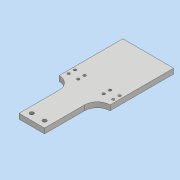
# Autodesk Inventor part: Wspornik pionowy osi Y
Saved by Autodesk Inventor 2018 (Build 220112000, 112)
## iProperties
Created: 2019-01-25
Part Number: Wspornik pionowy osi Y
Material: Ogólny
Document SubType Name: Modeling
Designer: Dawid
Density: 1 g/cm^3
Appearance: Domyślna
Author: Dawid
Autodesk Inventor part; units mm, degrees
ref_plane "YZ Plane" through (0, 0, 0) normal (1, 0, 0) x (0, 1, 0)
ref_plane "XZ Plane" through (0, 0, 0) normal (0, 1, 0) x (-1, 0, 0)
ref_plane "XY Plane" through (0, 0, 0) normal (0, 0, 1) x (1, 0, 0)
sketch "Szkic1" plane through (0, 0, 0) normal (0, 0, 1) x (1, 0, 0)
  line L0 (0, 0) -> (20, 0)
  line L1 (0, 0) -> (-20, 0)
  line L2 (-20, 0) -> (-20, 20)
  line L3 (-20, 0) -> (0, 0) construction
  line L4 (-20, 20) -> (20, 20)
  line L5 (20, 20) -> (20, 0)
  line L6 (-20, 0) -> (-20, 88)
  line L7 (-20, 88) -> (20, 88)
  line L8 (20, 88) -> (20, 20)
  line L9 (20, 88) -> (20, 93)
  line L10 (20, 93) -> (-20, 93)
  line L11 (-20, 93) -> (-20, 88)
  line L12 (0, 93) -> (35, 93)
  line L13 (35, 93) -> (40, 93)
  line L14 (0, 93) -> (-35, 93)
  line L15 (-35, 93) -> (-40, 93)
  line L16 (-40, 93) -> (-40, 103)
  line L17 (-40, 103) -> (40, 103)
  line L18 (40, 103) -> (40, 93)
  line L19 (-35, 93) -> (-35, 103)
  line L20 (35, 93) -> (35, 103)
  circle A0 centre (-35, 103) radius 1.5
  circle A1 centre (-35, 93) radius 1.5
  circle A2 centre (35, 103) radius 1.5
  circle A3 centre (35, 93) radius 1.5
  line L21 (40, 93) -> (40, 83)
  line L22 (40, 83) -> (20, 83)
  line L23 (-40, 93) -> (-40, 83)
  line L24 (-40, 83) -> (-20, 83)
  line L25 (-40, 103) -> (-40, 183)
  line L26 (40, 103) -> (40, 183)
  line L27 (40, 183) -> (-40, 183)
  dimension "d0" = 20
  dimension "d1" = 20
  dimension "d2" = 20
  dimension "d3" = 90
  dimension "d4" = 88
  dimension "d5" = 5
  dimension "d6" = 35
  dimension "d7" = 5
  dimension "d8" = 35
  dimension "d9" = 5
  dimension "d10" = 10
  dimension "d11" = 3
  dimension "d12" = 3
  dimension "d13" = 3
  dimension "d14" = 3
  dimension "d15" = 10
  dimension "d16" = 10
  dimension "d17" = 80
  dimension "d18" = 80
  constraints: 56 end point, 11 perpendicular, 9 point on line, 6 vertical, 5 horizontal, 4 centre point, 4 coincident, 1 midpoint, 1 parallel
  measures "d0" distance of L0.start L0.end
  measures "d1" distance of L0.start L1.end
  measures "d2" distance of L1.end L2.end
  measures "d3" angle of L3 L2
  measures "d4" distance of L1.end L6.end
  measures "d5" distance of L7.end L9.end
  measures "d6" distance of L12.start L12.end
  measures "d7" distance of L12.end L13.end
  measures "d8" distance of L12.start L14.end
  measures "d9" distance of L14.end L15.end
  measures "d10" distance of L15.end L16.end
  measures "d11" diameter of A0
  measures "d12" diameter of A1
  measures "d13" diameter of A2
  measures "d14" diameter of A3
  measures "d15" distance of L13.end L21.end
  measures "d16" distance of L15.end L23.end
  measures "d17" distance of L16.end L25.end
  measures "d18" distance of L17.end L26.end
extrude "Wyciągnięcie proste1" add sketch "Szkic1" along normal blind 8
sketch "Szkic2" plane through (0, 0, 8) normal (0, 0, 1) x (1, 0, 0)
  circle A0 centre (-35, 103) radius 1.5 projected
  circle A1 centre (-35, 93) radius 1.5 projected
  circle A2 centre (35, 103) radius 1.5 projected
  circle A3 centre (35, 93) radius 1.5 projected
  line L0 (-35, 103) -> (35, 103)
  line L1 (-35, 93) -> (35, 93)
  line L2 (-35, 103) -> (-20, 103)
  line L3 (-20, 103) -> (-20, 93)
  line L4 (35, 103) -> (20, 103)
  line L5 (20, 103) -> (20, 93)
  circle A4 centre (-20, 103) radius 2
  circle A5 centre (-20, 93) radius 2
  circle A6 centre (20, 103) radius 2
  circle A7 centre (20, 93) radius 2
  line L6 (40, 83) -> (40, 183) projected
  line L7 (40, 183) -> (-40, 183) projected
  line L8 (-40, 183) -> (-40, 83) projected
  line L9 (-40, 83) -> (-20, 83) projected
  line L10 (-20, 83) -> (-20, 0) projected
  line L11 (-20, 0) -> (20, 0) projected
  line L12 (20, 0) -> (20, 83) projected
  line L13 (20, 83) -> (40, 83) projected
  line L14 (-20, 0) -> (20, 0) projected
  line L15 (-20, 0) -> (-20, 10)
  line L16 (-20, 83) -> (-20, 0) projected
  line L17 (-20, 10) -> (20, 10)
  line L18 (-20, 10) -> (-10, 10)
  line L19 (20, 10) -> (10, 10)
  circle A8 centre (-10, 10) radius 3
  circle A9 centre (10, 10) radius 3
  point P0 (0, 0)
  dimension "d21" = 15
  dimension "d22" = 15
  dimension "d23" = 4
  dimension "d24" = 4
  dimension "d25" = 4
  dimension "d26" = 4
  dimension "d27" = 10
  dimension "d28" = 10
  dimension "d29" = 10
  dimension "d30" = 6
  dimension "d31" = 6
  constraints: 20 end point, 8 point on line, 6 centre point, 6 coincident, 3 perpendicular, 2 horizontal
  measures "d21" distance of L0.start L2.end
  measures "d22" distance of L0.end L4.end
  measures "d23" diameter of A4
  measures "d24" diameter of A5
  measures "d25" diameter of A6
  measures "d26" diameter of A7
  measures "d27" distance of L10.end L15.end
  measures "d28" distance of L15.end L18.end
  measures "d29" distance of L17.end L19.end
  measures "d30" diameter of A8
  measures "d31" diameter of A9
hole "Otwór1" at (-20, 103, 8) at (-20, 93, 8) at (20, 103, 8) at (20, 93, 8) at (-35, 103, 8) at (-35, 93, 8) at (35, 103, 8) at (35, 93, 8) direction (0, 0, -1) diameter 4 end through all
sketch "Szkic3" plane through (0, 0, 8) normal (0, 0, 1) x (1, 0, 0)
  circle A0 centre (-10, 10) radius 3 projected
  circle A1 centre (10, 10) radius 3 projected
  point P0 (0, 0)
hole "Otwór2" at (-10, 10, 8) at (10, 10, 8) direction (0, 0, -1) diameter 6 end through all
fillet "Zaokrąglenie1" radius 20 2 edges at (20, 83, 4) (-20, 83, 4)
